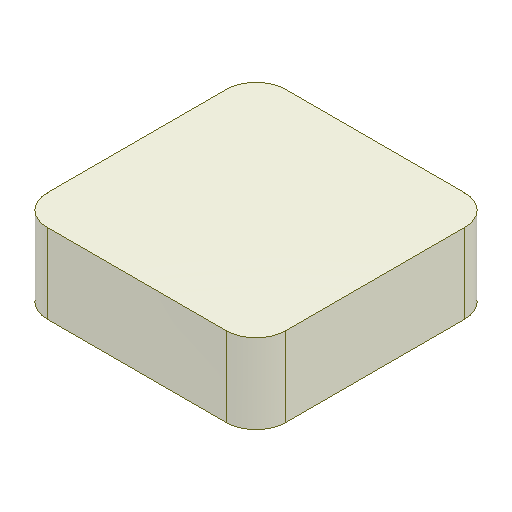
# Autodesk Inventor part: 3DP_TPU_Rubber_Feet
Saved by Autodesk Inventor 2026.1 (Build 301233000, 233)
## iProperties
Created: 2016-08-19
Part Number: 3DP_TPU_Rubber_Feet
Material: Ogólny
Document SubType Name: Modeling
Designer: Andrzej
Density: 1 g/cm^3
Appearance: Smooth - Ivory
Author: Andrzej
Autodesk Inventor part; units mm, degrees
ref_plane "YZ Plane" through (0, 0, 0) normal (1, 0, 0) x (0, 1, 0)
ref_plane "XZ Plane" through (0, 0, 0) normal (0, 1, 0) x (-1, 0, 0)
ref_plane "XY Plane" through (0, 0, 0) normal (0, 0, 1) x (1, 0, 0)
sketch "Szkic1" plane through (0, 0, 0) normal (0, 0, 1) x (1, 0, 0)
  arc A0 (-13.5, 15) -> (-15, 13.5) centre (-13.5, 13.5) ccw
  line L0 (-15, 13.5) -> (-15, -13.5)
  arc A1 (-15, -13.5) -> (-13.5, -15) centre (-13.5, -13.5) ccw
  line L1 (-13.5, -15) -> (13.5, -15)
  arc A2 (13.5, -15) -> (15, -13.5) centre (13.5, -13.5) ccw
  line L2 (15, -13.5) -> (15, 13.5)
  arc A3 (15, 13.5) -> (13.5, 15) centre (13.5, 13.5) ccw
  line L3 (13.5, 15) -> (-13.5, 15)
  arc A4 (-13.5, 18) -> (-18, 13.5) centre (-13.5, 13.5) ccw
  line L4 (-18, 13.5) -> (-18, -13.5)
  arc A5 (-18, -13.5) -> (-13.5, -18) centre (-13.5, -13.5) ccw
  line L5 (-13.5, -18) -> (13.5, -18)
  arc A6 (13.5, -18) -> (18, -13.5) centre (13.5, -13.5) ccw
  line L6 (18, -13.5) -> (18, 13.5)
  arc A7 (18, 13.5) -> (13.5, 18) centre (13.5, 13.5) ccw
  line L7 (13.5, 18) -> (-13.5, 18)
  dimension "d0" = 3
  constraints: 16 end point, 16 point on circle, 8 centre point, 7 other
  measures "d0" distance between parallel lines of L3 L7
extrude "Wyciągnięcie proste1" add sketch "Szkic1" along normal blind 4 contours L3 A3 L2 A2 L1 A1 L0 A0 | L7 A7 L6 A6 L5 A5 L4 A4
extrude "Wyciągnięcie proste2" add sketch "Szkic1" against normal blind 8
